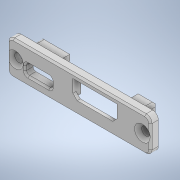
# Autodesk Inventor part: cover
Saved by Autodesk Inventor 2021 (Build 250183000, 183)
## iProperties
Created: 2026-06-25
Part Number: cover
Material: Generic
Document SubType Name: Modeling
Designer: Toby
Density: 1 g/cm^3
Appearance: Default
Author: Toby
Autodesk Inventor part; units mm, degrees
ref_plane "YZ Plane" through (0, 0, 0) normal (1, 0, 0) x (0, 1, 0)
ref_plane "XZ Plane" through (0, 0, 0) normal (0, 1, 0) x (-1, 0, 0)
ref_plane "XY Plane" through (0, 0, 0) normal (0, 0, 1) x (1, 0, 0)
sketch "Sketch1" plane through (0, 0, 0) normal (0, 0, 1) x (1, 0, 0)
  line L0 (-21.6, 6) -> (21.6, 6)
  line L1 (21.6, 6) -> (21.6, -6)
  line L2 (21.6, -6) -> (-21.6, -6)
  line L3 (-21.6, -6) -> (-21.6, 6)
  point P0 (0, 0)
  dimension "d0" = 43.2
  dimension "d1" = 12
  dimension "d2" = 6
  dimension "d3" = 21.6
  constraints: 8 end point, 2 parallel, 1 horizontal, 1 perpendicular
  measures "d0" distance of L0.start L0.end
  measures "d1" distance of L2.end L0.start
  measures "d2" distance from line of point (0, 0) L0
  measures "d3" distance from line of point (0, 0) L3
extrude "Extrusion1" add sketch "Sketch1" along normal blind 2.8
sketch "Sketch2" plane through (0, 0, 2.8) normal (0, 0, 1) x (1, 0, 0)
  line L0 (-18.9, 0.8) -> (-9.6, 0.8)
  line L1 (-9.6, 0.8) -> (-9.6, -2.8)
  line L2 (-9.6, -2.8) -> (-18.9, -2.8)
  line L3 (-18.9, -2.8) -> (-18.9, 0.8)
  line L4 (-21.6, -6) -> (21.6, -6) projected
  line L5 (-21.6, 6) -> (-21.6, -6) projected
  point P0 (0, 0)
  dimension "d6" = 9.3
  dimension "d7" = 3.6
  dimension "d8" = 3.2
  dimension "d9" = 2.7
  constraints: 8 end point, 2 parallel, 1 horizontal, 1 perpendicular
  measures "d6" distance of L0.start L0.end
  measures "d7" distance of L2.end L0.start
  measures "d8" distance between parallel lines of L4 L2
  measures "d9" distance between parallel lines of L5 L3
extrude "Extrusion2" cut sketch "Sketch2" against normal blind 3
fillet "Fillet2" radius 1 4 edges at (-18.9, 0.8, 1.4) (-18.9, -2.8, 1.4) (-9.6, -2.8, 1.4) (-9.6, 0.8, 1.4)
sketch "Sketch5" plane through (0, 0, 2.8) normal (0, 0, 1) x (1, 0, 0)
  line L0 (-2.1, 4.4) -> (13.4, 4.4)
  line L1 (13.4, 4.4) -> (13.4, -1.6)
  line L2 (13.4, -1.6) -> (-2.1, -1.6)
  line L3 (-2.1, -1.6) -> (-2.1, 4.4)
  line L4 (21.6, -6) -> (21.6, 6) projected
  line L5 (21.6, 6) -> (-21.6, 6) projected
  point P0 (0, 0)
  point P1 (21.6, -4)
  point P2 (21.6, 4)
  point P3 (19.6, 6)
  point P4 (-5.1, 6)
  dimension "d36" = 6
  dimension "d37" = 15.5
  dimension "d38" = 8.2
  dimension "d39" = 1.6
  constraints: 8 end point, 2 parallel, 1 horizontal, 1 perpendicular
  measures "d36" distance of L2.end L0.start
  measures "d37" distance of L0.start L0.end
  measures "d38" distance between parallel lines of L4 L1
  measures "d39" distance between parallel lines of L5 L0
extrude "Extrusion4" cut sketch "Sketch5" against normal blind 3
chamfer "Chamfer3" distance 1.5 angle 45 2 edges at (-2.1, -1.6, 1.4) (13.4, -1.6, 1.4)
sketch "Sketch6" plane through (0, 0, 0) normal (0, 0, -1) x (-1, 0, 0)
  line L0 (-17.1, -1.6) -> (5.9, -1.6)
  line L1 (5.9, -1.6) -> (5.9, -5.2)
  line L2 (5.9, -5.2) -> (-17.1, -5.2)
  line L3 (-17.1, -5.2) -> (-17.1, -1.6)
  line L4 (-13.4, -0.1) -> (-13.4, 4.4) projected
  line L5 (2.1, 4.4) -> (2.1, -0.1) projected
  line L6 (-13.4, 4.4) -> (2.1, 4.4) projected
  point P0 (0, 0)
  dimension "d45" = 3.7
  dimension "d46" = 3.8
  dimension "d48" = 3.6
  dimension "d50" = 9.6
  constraints: 6 end point, 1 horizontal, 1 parallel, 1 vertical, 3 other
  measures "d45" distance between parallel lines of L3 L4
  measures "d46" distance between parallel lines of L1 L5
  measures "d50" distance between parallel lines of L2 L6
extrude "Extrusion5" cut sketch "Sketch6" against normal blind 1.7
sketch "Sketch7" plane through (0, 0, 0) normal (0, 0, -1) x (-1, 0, 0)
  line L0 (-13.4, -0.1) -> (-13.4, 4.4) projected
  line L1 (5.9, -5.2) -> (-17.1, -5.2) projected
  line L2 (-13.4, 4.4) -> (2.1, 4.4)
  line L3 (2.1, 4.4) -> (2.1, -5.2)
  line L4 (2.1, -5.2) -> (-13.4, -5.2)
  line L5 (-13.4, -5.2) -> (-13.4, 4.4)
  line L6 (2.1, 4.4) -> (2.1, -0.1) projected
  point P0 (0, 0)
  constraints: 8 end point, 2 parallel, 1 collinear, 1 horizontal, 1 perpendicular, 1 point on line
extrude "Extrusion6" cut sketch "Sketch7" against normal blind 1.7
chamfer "Chamfer4" distance 1.7 angle 45 1 edges at (5.6, -5.2, 1.7)
sketch "Sketch9" plane through (0, 0, 0) normal (0, 0, -1) x (-1, 0, 0)
  line L0 (10, 4.4) -> (20, 4.4)
  line L1 (20, 4.4) -> (20, 2.4)
  line L2 (20, 2.4) -> (10, 2.4)
  line L3 (10, 2.4) -> (10, 4.4)
  line L4 (-21.6, 6) -> (21.6, 6) projected
  line L5 (21.6, 6) -> (21.6, -6) projected
  point P0 (0, 0)
  point P1 (-19.6, 6)
  point P2 (19.6, 6)
  point P3 (21.6, 4)
  point P4 (21.6, -4)
  dimension "d58" = 1.6
  dimension "d59" = 1.6
  dimension "d60" = 2
  dimension "d61" = 10
  constraints: 8 end point, 2 parallel, 1 horizontal, 1 perpendicular
  measures "d58" distance between parallel lines of L4 L0
  measures "d59" distance between parallel lines of L5 L1
  measures "d60" distance between parallel lines of L0 L2
  measures "d61" distance between parallel lines of L1 L3
extrude "Extrusion7" add sketch "Sketch9" along normal blind 5
chamfer "Chamfer5" distance 1 angle 45 2 edges at (-10, 3.4, -5) (-20, 3.4, -5)
fillet "Fillet4" radius 1 1 edges at (-15, 2.4, 0)
sketch "Sketch10" plane through (0, 0, 0) normal (0, 0, -1) x (-1, 0, 0)
  line L0 (-20, 4.4) -> (-14, 4.4)
  line L1 (-14, 4.4) -> (-14, 2.4)
  line L2 (-14, 2.4) -> (-20, 2.4)
  line L3 (-20, 2.4) -> (-20, 4.4)
  line L4 (-21.6, 6) -> (21.6, 6) projected
  line L5 (-21.6, -6) -> (-21.6, 6) projected
  point P0 (0, 0)
  point P1 (-19.6, 6)
  point P2 (19.6, 6)
  point P3 (-21.6, -4)
  point P4 (-21.6, 4)
  dimension "d68" = 1.6
  dimension "d69" = 1.6
  dimension "d70" = 2
  dimension "d71" = 6
  constraints: 8 end point, 2 parallel, 1 horizontal, 1 perpendicular
  measures "d68" distance between parallel lines of L0 L4
  measures "d69" distance between parallel lines of L5 L3
  measures "d70" distance between parallel lines of L2 L0
  measures "d71" distance between parallel lines of L3 L1
extrude "Extrusion8" add sketch "Sketch10" along normal blind 5
sketch "Sketch11" plane through (0, 0, 0) normal (0, 0, -1) x (-1, 0, 0)
  line L0 (-20, 4.4) -> (-20, 2.4) projected
  line L1 (-20, 2.4) -> (-18, 2.4)
  line L2 (-18, 2.4) -> (-18, -4.4)
  line L3 (-18, -4.4) -> (-20, -4.4)
  line L4 (-20, -4.4) -> (-20, 2.4)
  line L5 (21.6, -6) -> (-21.6, -6) projected
  point P0 (0, 0)
  point P1 (19.6, -6)
  point P2 (-19.6, -6)
  dimension "d78" = 2
  dimension "d79" = 1.6
  constraints: 8 end point, 2 parallel, 1 horizontal, 1 perpendicular
  measures "d78" distance between parallel lines of L4 L2
  measures "d79" distance between parallel lines of L5 L3
extrude "Extrusion9" add sketch "Sketch11" along normal blind 5
chamfer "Chamfer7" distance 1 angle 45 2 edges at (20, 0, -5) (17, 4.4, -5)
chamfer "Chamfer8" distance 1 angle 45 1 edges at (-15, 4.4, -5)
fillet "Fillet6" radius 1 1 edges at (20, 4.4, -2)
fillet "Fillet7" radius 1 1 edges at (-20, 4.4, -2)
fillet "Fillet8" radius 1 1 edges at (20, -4.4, -2)
sketch "Sketch12" plane through (0, 0, 2.8) normal (0, 0, 1) x (1, 0, 0)
  line L0 (-21.6, 6) -> (-21.6, -6) projected
  line L1 (-21.6, 6) -> (-25.1, 6)
  line L2 (-25.1, 6) -> (-25.1, -6)
  line L3 (-25.1, -6) -> (-21.6, -6)
  line L4 (-21.6, -6) -> (-21.6, 6)
  line L5 (21.6, -6) -> (21.6, 6) projected
  line L6 (21.6, 6) -> (25.1, 6)
  line L7 (25.1, 6) -> (25.1, -6)
  line L8 (25.1, -6) -> (21.6, -6)
  line L9 (21.6, -6) -> (21.6, 6)
  line L10 (-21.6, -6) -> (21.6, -6) projected
  point P0 (0, 0)
  dimension "d91" = 3.5
  dimension "d92" = 3.5
  constraints: 16 end point, 4 parallel, 2 horizontal, 2 perpendicular, 1 collinear, 1 point on line
  measures "d91" distance between parallel lines of L0 L2
  measures "d92" distance between parallel lines of L5 L7
extrude "Extrusion10" add sketch "Sketch12" against normal blind 2.8
fillet "Fillet9" radius 2 4 edges at (-25.1, 6, 1.4) (-25.1, -6, 1.4) (25.1, 6, 1.4) (25.1, -6, 1.4)
sketch "Sketch13" plane through (0, 0, 2.8) normal (0, 0, 1) x (1, 0, 0)
  line L0 (-25.1, 4) -> (-25.1, -4) projected
  line L1 (25.1, -4) -> (25.1, 4) projected
  point P0 (0, 0)
  point P1 (-22.3, 0)
  point P2 (22.3, 0)
  dimension "d96" = 2.8
  dimension "d97" = 2.8
  measures "d96" distance from line of L0 point (-22.3, 0)
  measures "d97" distance from line of L1 point (22.3, 0)
hole "Hole2" at (-22.3, 0, 2.8) at (22.3, 0, 2.8) direction (0, 0, -1) diameter 3 depth 8 tip angle 118 countersink diameter 5.5 countersink angle 90
chamfer "Chamfer9" distance 0.6 angle 45 8 edges at (0, 6, 2.8) (-24.5142, 5.4142, 2.8) (-25.1, 0, 2.8) (-24.5142, -5.4142, 2.8) (0, -6, 2.8) (24.5142, -5.4142, 2.8) (25.1, 0, 2.8) (24.5142, 5.4142, 2.8)
chamfer "Chamfer10" distance 0.6 angle 45 8 edges at (-14.25, 0.8, 2.8) (-9.8929, 0.5071, 2.8) (-9.6, -1, 2.8) (-9.8929, -2.5071, 2.8) (-14.25, -2.8, 2.8) (-18.6071, -2.5071, 2.8) (-18.9, -1, 2.8) (-18.6071, 0.5071, 2.8)
body "Solid1"
